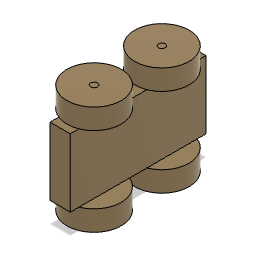
henosv0309v1 (Autodesk Fusion 360 design; units mm, degrees)
Autodesk Fusion 360 part; units mm, degrees
sketch "草图1" plane through (0, 0, 0) normal (1, 0, 0) x (0, 0, -1) in component "body"
  line L0 (0, 0) -> (-100, 0)
  line L1 (-100, 0) -> (-100, 50)
  line L2 (-100, 50) -> (0, 50)
  line L3 (0, 50) -> (0, 0)
  dimension "d11" = 100
  dimension "d12" = 50
  constraint horizontal L0
  constraint vertical L1
  constraint horizontal L2
  constraint vertical L3
  constraint coincident L0.start L3.end
  measures "d11" distance of L0.start L0.end
  measures "d12" distance of L0.start L2.end
extrude "拉伸1" add sketch "草图1" along normal blind 15 makes body 1 in component "body"
sketch "草图1 (2)" plane through (0, 50, 0) normal (0, 1, 0) x (-1, 0, 0) in component "axis"
  line L0 (0, 0) -> (0, 100)
  line L1 (0, 100) -> (-15, 100)
  line L2 (-15, 100) -> (-15, 0)
  line L3 (-15, 0) -> (0, 0)
  circle A0 centre (-7.5, 25) radius 2.5
  line L4 (0, 50) -> (-46.2077, 50)
  circle A1 centre (-7.5, 75) radius 2.5
  dimension "d15" = 5
  dimension "d16" = 25
  dimension "d17" = 7.5
  constraint midpoint L0 L4.start
  constraint perpendicular L0 L4
  constraint symmetric A0 L4 A1
  measures "d15" diameter of A0
  measures "d16" distance of A0.centre L4
  measures "d17" distance of L0 A0.centre
extrude "拉伸1'" add sketch "草图1 (2)" along normal blind 15 and the other way blind 65 separate body contours A0 | A1 makes body 2 at (5.0124, 28.3333, 24.7511) makes body 3 at (5.0124, 28.3333, 74.7511) in component "axis"
sketch "草图2" plane through (0, 0, 0) normal (0, -1, 0) x (1, 0, 0)
  line L0 (0, 100) -> (0, 0)
  line L1 (0, 0) -> (15, 0)
  line L2 (15, 0) -> (15, 100)
  line L3 (15, 100) -> (0, 100)
  circle A0 centre (-67.2818, 39.9129) radius 20
  dimension "d26" = 40
  measures "d26" diameter of A0
extrude "拉伸2" add sketch "草图2" along normal blind 15 separate body contours A0 makes body 4
copy_body "实体->零部件1" bodies 4 removing the originals makes body 5 in component "wheel"
component "body" placed x (1, 0, 0) y (0, -1, 0) z (0, 0, -1) at (-74.7818, -15, 114.9129)
component "axis" placed x (1, 0, 0) y (0, -1, 0) z (0, 0, -1) at (-74.7818, -15, 114.9129)
component "wheel" placed x (1, 0, 0) y (0, 1, 0) z (0, 0, 1) at (0, 0, 0)
component "wheel" placed x (1, 0, 0) y (0, -1, 0) z (0, 0, -1) at (0, -80, 79.8258)
component "wheel" placed x (1, 0, 0) y (0, -1, 0) z (0, 0, -1) at (0, -80, 129.8258)
component "wheel" placed x (1, 0, 0) y (0, 1, 0) z (0, 0, 1) at (0, 0, 50)
equation "length = 100 mm"
equation "width = 50 mm"
equation "thickness = 15 mm"
equation "wheelDistance = 50 mm"
equation "wheelDiameter = 40 mm"
equation "wheelThickness = 15 mm"
equation "d11 = length"
equation "d12 = width"
equation "d13 = thickness"
equation "d16 = length / 4"
equation "d17 = thickness / 2"
equation "d18 = wheelThickness"
equation "d20 = wheelThickness + width"
equation "d24 = length / 4"
equation "d25 = wheelThickness"
equation "d26 = wheelDiameter"
equation "d27 = wheelThickness"
equation "d31 = 0.25 * length"
equation "d32 = wheelDistance / 2 - width / 2"
equation "d35 = -0.25 * length"
equation "d36 = wheelDistance / 2 - width / 2"
equation "d39 = 0.25 * length"
equation "d40 = wheelDistance / 2 - width / 2"
equation "d43 = -0.25 * length"
equation "d44 = wheelDistance / 2 - width / 2"
